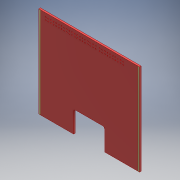
# Autodesk Inventor part: CardRCS_PCB
Saved by Autodesk Inventor 2017 (Build 210142000, 142)
## iProperties
Created: 2017-10-19
Part Number: CardRCS_PCB
Material: Epoxy Resin
Document SubType Name: Modeling
Designer: Bradley
Density: 1.14 g/cm^3
Appearance: Smooth - Red
Author: Bradley
Autodesk Inventor part; units mm, degrees
ref_plane "YZ Plane" through (0, 0, 0) normal (1, 0, 0) x (0, 1, 0)
ref_plane "XZ Plane" through (0, 0, 0) normal (0, 1, 0) x (-1, 0, 0)
ref_plane "XY Plane" through (0, 0, 0) normal (0, 0, 1) x (1, 0, 0)
sketch "Sketch1" plane through (0, 0, 0) normal (0, 1, 0) x (-1, 0, 0)
  line L0 (-48.7, 6.1) -> (48.7, 6.1)
  line L1 (48.7, 6.1) -> (48.7, -81.9)
  line L2 (48.7, -81.9) -> (-48.7, -81.9)
  line L3 (-48.7, -81.9) -> (-48.7, 6.1)
  point P0 (0, 0)
  point P1 (0, 6.1)
  dimension "d0" = 88
  dimension "d1" = 97.4
  dimension "d24" = 6.1
  constraints: 8 end point, 2 parallel, 1 horizontal, 1 midpoint, 1 perpendicular, 1 vertical alignment
  measures "d0" distance of L0.end L1.end
  measures "d1" distance of L0.start L0.end
  measures "d24" distance from line of point (0, 0) L0
extrude "Extrusion1" add sketch "Sketch1" along normal mid plane 1.6
sketch "Sketch2" plane through (0, 0.8, 0) normal (0, 1, 0) x (1, 0, 0)
  line L0 (-48.7, -6.1) -> (48.7, -6.1) projected
  line L1 (48.7, -6.1) -> (48.7, 81.9) projected
  line L2 (48.7, 81.9) -> (-48.7, 81.9) projected
  line L3 (-48.7, 81.9) -> (-48.7, -6.1) projected
  line L4 (-48.7, -6.1) -> (48.7, -6.1) projected
  line L5 (48.7, 81.9) -> (-48.7, 81.9) projected
  line L6 (-46.8, -6.1) -> (46.8, -6.1)
  line L7 (46.8, -6.1) -> (46.8, 81.9)
  line L8 (46.8, 81.9) -> (-46.8, 81.9)
  line L9 (-46.8, 81.9) -> (-46.8, -6.1)
  point P0 (0, 0)
  point P1 (0, 81.9)
  point P2 (0, 81.9)
  dimension "d4" = 93.6
  constraints: 8 end point, 4 midpoint, 2 parallel, 2 point on line, 1 horizontal, 1 perpendicular
  measures "d4" distance between parallel lines of L7 L9
split_face "Split1"
sketch "Sketch3" plane through (-46.8, 0.8, -81.9) normal (0, 1, 0) x (1, 0, 0)
  line L0 (93.6, 0) -> (93.6, -88) projected
  line L1 (93.6, 0) -> (0, 0) projected
  line L2 (0, -88) -> (0, 0) projected
  line L3 (0, -88) -> (93.6, -88) projected
  point P0 (46.8, -81.9)
  point P1 (4.8, -84.44)
  point P2 (30.2, -84.44)
  point P3 (56.87, -84.44)
  point P4 (56.87, -81.9)
  point P5 (30.2, -81.9)
  point P6 (4.8, -81.9)
  point P7 (59.41, -84.44)
  point P8 (32.74, -84.44)
  point P9 (7.34, -84.44)
  point P10 (59.41, -81.9)
  point P11 (32.74, -81.9)
  point P12 (7.34, -81.9)
  point P13 (61.95, -84.44)
  point P14 (35.28, -84.44)
  point P15 (9.88, -84.44)
  point P16 (61.95, -81.9)
  point P17 (35.28, -81.9)
  point P18 (9.88, -81.9)
  point P19 (64.49, -84.44)
  point P20 (37.82, -84.44)
  point P21 (12.42, -84.44)
  point P22 (64.49, -81.9)
  point P23 (37.82, -81.9)
  point P24 (12.42, -81.9)
  point P25 (67.03, -84.44)
  point P26 (40.36, -84.44)
  point P27 (14.96, -84.44)
  point P28 (67.03, -81.9)
  point P29 (40.36, -81.9)
  point P30 (14.96, -81.9)
  point P31 (69.57, -84.44)
  point P32 (42.9, -84.44)
  point P33 (17.5, -84.44)
  point P34 (69.57, -81.9)
  point P35 (42.9, -81.9)
  point P36 (17.5, -81.9)
  point P37 (72.11, -84.44)
  point P38 (45.44, -84.44)
  point P39 (20.04, -84.44)
  point P40 (72.11, -81.9)
  point P41 (45.44, -81.9)
  point P42 (20.04, -81.9)
  point P43 (74.65, -84.44)
  point P44 (47.98, -84.44)
  point P45 (22.58, -84.44)
  point P46 (74.65, -81.9)
  point P47 (47.98, -81.9)
  point P48 (22.58, -81.9)
  point P49 (77.19, -84.44)
  point P50 (50.52, -84.44)
  point P51 (25.12, -84.44)
  point P52 (77.19, -81.9)
  point P53 (50.52, -81.9)
  point P54 (25.12, -81.9)
  point P55 (79.73, -84.44)
  point P56 (53.06, -84.44)
  point P57 (27.66, -84.44)
  point P58 (79.73, -81.9)
  point P59 (53.06, -81.9)
  point P60 (27.66, -81.9)
  dimension "d7" = 2.54
  dimension "d10" = 2.54
  dimension "d13" = 25.4
  dimension "d14" = 52.07
  dimension "d15" = 42
  dimension "d16" = 6.1
  constraints: 2 horizontal alignment, 1 horizontal, 1 vertical, 57 other
  measures "d7" distance of point (56.87, -84.44) point (56.87, -81.9)
  measures "d10" distance of point (56.87, -84.44) point (59.41, -84.44)
  measures "d13" distance of point (30.2, -84.44) point (4.8, -84.44)
  measures "d14" distance of point (56.87, -84.44) point (4.8, -84.44)
  measures "d15" distance of point (46.8, -81.9) point (4.8, -81.9)
  measures "d16" distance from line of point (4.8, -81.9) L3
hole "Hole1" at (-42, 0.8, 2.54) at (-16.6, 0.8, 2.54) at (10.07, 0.8, 2.54) at (10.07, 0.8, 0) at (-16.6, 0.8, 0) at (-42, 0.8, 0) at (12.61, 0.8, 2.54) at (-14.06, 0.8, 2.54) at (-39.46, 0.8, 2.54) at (12.61, 0.8, 0) at (-14.06, 0.8, 0) at (-39.46, 0.8, 0) at (15.15, 0.8, 2.54) at (-11.52, 0.8, 2.54) at (-36.92, 0.8, 2.54) at (15.15, 0.8, 0) at (-11.52, 0.8, 0) at (-36.92, 0.8, 0) at (17.69, 0.8, 2.54) at (-8.98, 0.8, 2.54) at (-34.38, 0.8, 2.54) at (17.69, 0.8, 0) at (-8.98, 0.8, 0) at (-34.38, 0.8, 0) at (20.23, 0.8, 2.54) at (-6.44, 0.8, 2.54) at (-31.84, 0.8, 2.54) at (20.23, 0.8, 0) at (-6.44, 0.8, 0) at (-31.84, 0.8, 0) at (22.77, 0.8, 2.54) at (-3.9, 0.8, 2.54) at (-29.3, 0.8, 2.54) at (22.77, 0.8, 0) at (-3.9, 0.8, 0) at (-29.3, 0.8, 0) at (25.31, 0.8, 2.54) at (-1.36, 0.8, 2.54) at (-26.76, 0.8, 2.54) at (25.31, 0.8, 0) at (-1.36, 0.8, 0) at (-26.76, 0.8, 0) at (27.85, 0.8, 2.54) at (1.18, 0.8, 2.54) at (-24.22, 0.8, 2.54) at (27.85, 0.8, 0) at (1.18, 0.8, 0) at (-24.22, 0.8, 0) at (30.39, 0.8, 2.54) at (3.72, 0.8, 2.54) direction (0, -1, 0) diameter 0.889 end through all and at (-21.68, 0.8, 2.54) (30.39, 0.8, 0) (3.72, 0.8, 0) (-21.68, 0.8, 0) (32.93, 0.8, 2.54) (6.26, 0.8, 2.54) (-19.14, 0.8, 2.54) (32.93, 0.8, 0) (6.26, 0.8, 0) (-19.14, 0.8, 0)
sketch "Sketch4" plane through (-46.8, 0.8, -81.9) normal (0, 1, 0) x (1, 0, 0)
  circle A0 centre (53.06, -81.9) radius 0.4445 projected
  circle A1 centre (27.66, -84.44) radius 0.4445 projected
  circle A2 centre (79.73, -84.44) radius 0.4445 projected
  circle A3 centre (50.52, -81.9) radius 0.4445 projected
  circle A4 centre (25.12, -84.44) radius 0.4445 projected
  circle A5 centre (77.19, -84.44) radius 0.4445 projected
  circle A6 centre (47.98, -81.9) radius 0.4445 projected
  circle A7 centre (22.58, -84.44) radius 0.4445 projected
  circle A8 centre (74.65, -84.44) radius 0.4445 projected
  circle A9 centre (45.44, -81.9) radius 0.4445 projected
  circle A10 centre (20.04, -84.44) radius 0.4445 projected
  circle A11 centre (72.11, -84.44) radius 0.4445 projected
  circle A12 centre (42.9, -81.9) radius 0.4445 projected
  circle A13 centre (17.5, -84.44) radius 0.4445 projected
  circle A14 centre (69.57, -84.44) radius 0.4445 projected
  circle A15 centre (40.36, -81.9) radius 0.4445 projected
  circle A16 centre (14.96, -84.44) radius 0.4445 projected
  circle A17 centre (67.03, -84.44) radius 0.4445 projected
  circle A18 centre (37.82, -81.9) radius 0.4445 projected
  circle A19 centre (12.42, -84.44) radius 0.4445 projected
  circle A20 centre (64.49, -84.44) radius 0.4445 projected
  circle A21 centre (35.28, -81.9) radius 0.4445 projected
  circle A22 centre (9.88, -84.44) radius 0.4445 projected
  circle A23 centre (61.95, -84.44) radius 0.4445 projected
  circle A24 centre (32.74, -81.9) radius 0.4445 projected
  circle A25 centre (7.34, -84.44) radius 0.4445 projected
  circle A26 centre (59.41, -84.44) radius 0.4445 projected
  circle A27 centre (30.2, -81.9) radius 0.4445 projected
  circle A28 centre (56.87, -84.44) radius 0.4445 projected
  circle A29 centre (4.8, -84.44) radius 0.4445 projected
  circle A30 centre (30.2, -84.44) radius 0.4445 projected
  circle A31 centre (56.87, -81.9) radius 0.4445 projected
  circle A32 centre (4.8, -81.9) radius 0.4445 projected
  circle A33 centre (32.74, -84.44) radius 0.4445 projected
  circle A34 centre (59.41, -81.9) radius 0.4445 projected
  circle A35 centre (7.34, -81.9) radius 0.4445 projected
  circle A36 centre (35.28, -84.44) radius 0.4445 projected
  circle A37 centre (61.95, -81.9) radius 0.4445 projected
  circle A38 centre (9.88, -81.9) radius 0.4445 projected
  circle A39 centre (37.82, -84.44) radius 0.4445 projected
  circle A40 centre (64.49, -81.9) radius 0.4445 projected
  circle A41 centre (12.42, -81.9) radius 0.4445 projected
  circle A42 centre (40.36, -84.44) radius 0.4445 projected
  circle A43 centre (67.03, -81.9) radius 0.4445 projected
  circle A44 centre (14.96, -81.9) radius 0.4445 projected
  circle A45 centre (42.9, -84.44) radius 0.4445 projected
  circle A46 centre (69.57, -81.9) radius 0.4445 projected
  circle A47 centre (17.5, -81.9) radius 0.4445 projected
  circle A48 centre (45.44, -84.44) radius 0.4445 projected
  circle A49 centre (72.11, -81.9) radius 0.4445 projected
  circle A50 centre (20.04, -81.9) radius 0.4445 projected
  circle A51 centre (47.98, -84.44) radius 0.4445 projected
  circle A52 centre (74.65, -81.9) radius 0.4445 projected
  circle A53 centre (22.58, -81.9) radius 0.4445 projected
  circle A54 centre (50.52, -84.44) radius 0.4445 projected
  circle A55 centre (77.19, -81.9) radius 0.4445 projected
  circle A56 centre (25.12, -81.9) radius 0.4445 projected
  circle A57 centre (53.06, -84.44) radius 0.4445 projected
  circle A58 centre (79.73, -81.9) radius 0.4445 projected
  circle A59 centre (27.66, -81.9) radius 0.4445 projected
  line L0 (93.6, 0) -> (93.6, -88) projected
  line L1 (93.6, 0) -> (0, 0) projected
  line L2 (0, -88) -> (0, 0) projected
  line L3 (0, -88) -> (93.6, -88) projected
  line L4 (93.6, 0) -> (0, 0) projected
  line L5 (31.8, 0) -> (31.8, -19)
  arc A60 (31.8, -19) -> (33.8, -21) centre (33.8, -19) ccw
  line L6 (33.8, -21) -> (59.8, -21)
  arc A61 (59.8, -21) -> (61.8, -19) centre (59.8, -19) ccw
  line L7 (61.8, -19) -> (61.8, 0)
  point P0 (46.8, -81.9)
  point P1 (46.8, -21)
  dimension "d25" = 30
  dimension "d26" = 2
  dimension "d27" = 21
  constraints: 6 end point, 4 point on circle, 4 tangent, 2 centre point, 2 perpendicular, 2 point on line, 1 equal radius, 1 midpoint, 1 vertical, 1 vertical alignment
  measures "d25" distance between parallel lines of L7 L5
  measures "d26" radius of A60
  measures "d27" distance between parallel lines of L6 L4
extrude "Extrusion2" cut sketch "Sketch4" against normal through all contours L7 A61 L6 A60 L5 L1
equation "\"d13\" = 10 * d10"
equation "\"d14\" = 20.5 * d10"
body "Solid1"
